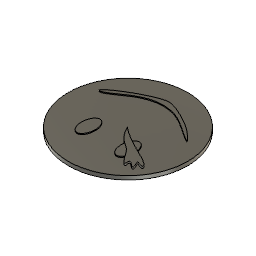
Comedian_Badge_v.1.0 (Autodesk Fusion 360 design; units mm, degrees)
part number: 2025-11-23-15-40-06-901
Autodesk Fusion 360 part; units mm, degrees
sketch "Sketch8" plane through (0, 0, 0) normal (0, 0, 1) x (1, 0, 0)
  circle A0 centre (0, 0) radius 73.66
  circle A1 centre (0, 0) radius 78.74
  arc A2 (-7.7116, -78.3615) -> (6.1475, -78.4997) centre (-0.7851, -78.7361) ccw
  arc A3 (-10.457, -78.213) -> (8.8953, -78.4059) centre (-0.7851, -78.7361) ccw
  dimension "d8" = 147.32
  dimension "d9" = 5.08
  dimension "d60" = 2.7495
  dimension "d61" = 78.7361
  dimension "d62" = 6.9366
  dimension "d63" = 0.5231
  constraint coincident A0.centre A1.centre
  constraint coincident A1 A2.centre
  constraint coincident A1 A2.start
  constraint coincident A1 A2.end
  measures "d8" diameter of A0
  measures "d61" vertical distance of A0.centre A2.centre
  measures "d62" radius of A2
  measures "d63" vertical distance of A2.centre A3.start
extrude "Inner Curve" add sketch "Sketch8" along normal blind 2.54 contours A0 makes body 1
extrude "Outer Curve" add sketch "Sketch8" along normal blind 5.08 from surface at -2.54 contours A1 bodies 1
sketch "Alignment 1" plane through (0, 0, 2.54) normal (0, 0, 1) x (-1, 0, 0)
  line L0 (0, 0) -> (52.0855, 52.0855) construction
  line L1 (0, 0) -> (-52.0855, 52.0855) construction
  line L2 (0, 0) -> (73.66, 0) construction
  line L3 (-26.0427, 26.0427) -> (26.0427, 26.0427) construction
  ellipse E0 centre (-26.0427, 26.0427) end of major axis (-26.0427, 41.2827) minor radius 8.89
  line L4 (-26.0427, 10.8027) -> (-26.0427, 41.2827) construction
  line L5 (-17.1527, 26.0427) -> (-34.9327, 26.0427) construction
  line L6 (0, 73.66) -> (0, -73.66) construction
  ellipse E1 centre (26.0427, 26.0427) end of major axis (26.0427, 41.2827) minor radius 8.89
  line L7 (0, 0) -> (0, -50.8) construction
  line L8 (34.9327, 26.0205) -> (34.9327, -64.8498) construction
  line L9 (-34.9327, 26.0427) -> (-34.9327, -64.2724) construction
  line L10 (-34.9327, -25.5899) -> (0, 0) construction
  line L11 (0, 0) -> (34.9327, -25.5899) construction
  circle A0 centre (0, 0) radius 78.74
  dimension "d16" = 73.66
  dimension "d17" = 135
  dimension "d18" = 73.66
  dimension "d19" = 30.48
  dimension "d20" = 17.78
  dimension "d23" = 50.8
  constraint coincident L0.start L1.start
  constraint horizontal L2
  constraint perpendicular L0 L1
  constraint midpoint L1 L3.start
  constraint midpoint L0 L3.end
  constraint coincident E0 L4.start
  constraint coincident E0 L4.end
  constraint coincident E0 L5.start
  constraint coincident E0 L5.end
  constraint coincident L3.start E0.centre
  constraint perpendicular L3 L4
  constraint perpendicular L2 L6
  constraint symmetric E0 L6 E1
  constraint coincident L3.end E1.centre
  constraint parallel L6 L7
  constraint coincident E1 L8.start
  constraint vertical L9
  constraint coincident L5.end L9.start
  constraint coincident L9 L10.start
  constraint symmetric L6 L10.start L11.end
  constraint coincident L8 L11.end
  measures "d16" distance of L0.start L0.end
  measures "d17" angle of L1 L2
  measures "d18" distance of L0.start L1.end
  measures "d19" distance of E0
  measures "d23" distance of L0.start L7.end
extrude "Eyes" add sketch "Alignment 1" along normal blind 1.27 contours E0 | E1 bodies 1
sketch "Alignment 2" plane through (0, 0, 2.54) normal (0, 0, 1) x (-1, 0, 0)
  ellipse E0 centre (26.0427, 26.0427) end of major axis (26.0427, 41.2827) minor radius 8.89
  ellipse E1 centre (-26.0427, 26.0427) end of major axis (-26.0427, 41.2827) minor radius 8.89
  line L0 (0.0807, 73.66) -> (0.0807, -73.66) construction
  line L1 (-34.9027, 24.7905) -> (-70.2813, -22.0531) construction
  line L2 (70.2813, -22.0531) -> (34.9327, 26.0427) construction
  line L3 (-70.2813, -22.0531) -> (70.2813, -22.0531) construction
  line L4 (70.2813, -22.0531) -> (-55.8551, -22.0531) construction
  line L5 (70.2813, -22.0531) -> (55.8541, -22.0531) construction
  circle A0 centre (0, 0) radius 78.74
  point P0 (70.2813, -22.0531)
  dimension "d25" = 140.5626
  dimension "d26" = 126.1364
  dimension "d27" = 14.4272
  dimension "d38" = 26.1235
  dimension "d40" = 37.062
  constraint vertical L0
  constraint coincident E1 L1.start
  constraint coincident E0 L2.end
  constraint horizontal L3
  constraint coincident P0 L2.start
  constraint parallel L3 L4
  constraint parallel L4 L5
  constraint horizontal E1.centre L2.end
  measures "d25" distance of L1.end P0
  measures "d26" distance of P0 L4.end
  measures "d27" distance of P0 L5.end
  measures "d38" distance of E1.centre L0
  measures "d40" angle of L0 L1
sketch "Blood Splatter" plane through (0, 0, 2.54) normal (0, 0, 1) x (-1, 0, 0)
  ellipse E0 centre (26.0427, 26.0427) end of major axis (26.0427, 41.2827) minor radius 8.89
  ellipse E1 centre (-26.0427, 26.0427) end of major axis (-26.0427, 41.2827) minor radius 8.89
  spline S0 degree 5 poles (0, 0) (0.1969, -0.2279) (0.5452, -0.589) (0.9093, -0.8334) (0.9612, -0.5275) (-0.05, 0.9191) (-2.4849, 3.3704) (-6.612, 6.7062) (-12.5588, 10.755) (-20.2217, 15.3044) (-29.241, 20.1083) (-38.8234, 24.9025) (-47.917, 29.3993) (-54.5396, 33.3328) (-57.6678, 36.3488) (-57.6761, 38.1034) (-55.5557, 38.4538) (-52.6453, 37.5711) (-50.0986, 36.1867) (-48.6444, 35.4193) (-48.5715, 36.1908) (-49.6251, 38.6476) (-51.0446, 41.8807) (-51.9382, 44.6253) (-51.5805, 45.747) (-49.7748, 44.8658) (-47.0902, 42.7681) (-44.4206, 40.7393) (-42.6094, 40.0043) (-42.0679, 41.1518) (-42.3499, 43.4995) (-42.6098, 45.7543) (-42.0762, 46.7002) (-40.6049, 45.9931) (-38.5035, 43.957) (-36.2304, 41.2005) (-34.0851, 38.2398) (-32.1418, 35.3844) (-30.3454, 32.8078) (-28.556, 30.5594) (-26.6153, 28.6009) (-24.4017, 26.8312) (-21.8967, 25.1168) (-19.1641, 23.3139) (-16.3177, 21.2902) (-13.4939, 18.9464) (-10.8205, 16.2389) (-8.3906, 13.1998) (-6.2268, 9.9645) (-4.3069, 6.7464) (-2.6019, 3.8005) (-1.4082, 1.8735) (-0.6359, 0.7782) (-0.1969, 0.2279) (0, 0) knots 0 0 0 0 0 0 0.02 0.04 0.06 0.08 0.1 0.12 0.14 0.16 0.18 0.2 0.22 0.24 0.26 0.28 0.3 0.32 0.34 0.36 0.38 0.4 0.42 0.44 0.46 0.48 0.5 0.52 0.54 0.56 0.58 0.6 0.62 0.64 0.66 0.68 0.7 0.72 0.74 0.76 0.78 0.8 0.82 0.84 0.86 0.88 0.9 0.92 0.94 0.96 0.98 1 1 1 1 1 1
  line L0 (-30.5379, 20.3586) -> (-61.7859, 36.9295)
  circle A0 centre (0, 0) radius 78.74
  point P0 (-46.1619, 28.644)
  point P1 (-53.9739, 37.8764)
  point P2 (-48.7659, 36.2193)
  point P3 (-51.3699, 45.215)
  point P4 (-42.8477, 40.4804)
  point P5 (-42.3742, 45.6884)
  point P6 (-37.6397, 42.8477)
  point P7 (-26.2768, 28.4073)
  point P8 (-10.416, 15.624)
  constraint coincident S0.start S0.end
  constraint midpoint P0 L0
extrude "Blood Splatter (1)" add sketch "Blood Splatter" along normal blind 2.54 separate body contours E1 S0 | E1 S0 | E1 S0 picked at (-25.5981, 21.049) picked at (-41.0519, 33.7718) picked at (-14.8563, 14.4402) makes body 2
sketch "Sketch18" plane through (0, 0, 2.54) normal (0, 0, 1) x (-1, 0, 0)
  spline S0 degree 5 poles (-55.9535, -21.9392) (-56.0022, -21.744) (-55.8793, -21.5301) (-55.0208, -21.7571) (-52.5792, -23.128) (-47.8442, -26.2124) (-42.0998, -30.0649) (-36.0544, -34.0423) (-30.3017, -37.604) (-25.1448, -40.4801) (-20.6388, -42.6257) (-16.6704, -44.1389) (-13.0259, -45.1898) (-9.4597, -45.9505) (-5.7724, -46.5104) (-1.8468, -46.8516) (2.3726, -46.8991) (6.8856, -46.5525) (11.6474, -45.7252) (16.5776, -44.3802) (21.5765, -42.5258) (26.5403, -40.2111) (31.3775, -37.5211) (36.0225, -34.5725) (40.457, -31.5086) (44.7078, -28.4957) (48.7877, -25.7179) (52.6437, -23.3733) (56.1063, -21.669) (58.8309, -20.8181) (60.2592, -21.0311) (59.9022, -22.4205) (57.6456, -24.8935) (53.6874, -28.2022) (48.4274, -32.0109) (42.3717, -35.9609) (36.0374, -39.7303) (29.8422, -43.1091) (24.0621, -46.0131) (18.8561, -48.4346) (14.2723, -50.4133) (10.2604, -51.9964) (6.6832, -53.2078) (3.3234, -54.0039) (-0.0891, -54.2677) (-3.8037, -53.8825) (-7.9919, -52.7801) (-12.6688, -51.0145) (-17.6745, -48.7761) (-22.7855, -46.2861) (-27.7875, -43.7268) (-32.5855, -41.1345) (-37.2462, -38.3635) (-42.2173, -34.8625) (-47.266, -30.8034) (-51.8146, -26.7345) (-54.4608, -24.0641) (-55.5866, -22.7015) (-55.9047, -22.1344) (-55.9535, -21.9392) knots 0 0 0 0 0 0 0.018182 0.036364 0.054545 0.072727 0.090909 0.109091 0.127273 0.145455 0.163636 0.181818 0.2 0.218182 0.236364 0.254545 0.272727 0.290909 0.309091 0.327273 0.345455 0.363636 0.381818 0.4 0.418182 0.436364 0.454545 0.472727 0.490909 0.509091 0.527273 0.545455 0.563636 0.581818 0.6 0.618182 0.636364 0.654545 0.672727 0.690909 0.709091 0.727273 0.745455 0.763636 0.781818 0.8 0.818182 0.836364 0.854545 0.872727 0.890909 0.909091 0.927273 0.945455 0.963636 0.981818 1 1 1 1 1 1
  line L0 (-23.2998, -46.7696) -> (-46.7696, -32.4836)
  point P0 (-35.2048, -34.5245)
  point P1 (-11.0546, -45.5791)
  point P2 (6.9729, -46.4295)
  point P3 (34.6946, -35.3748)
  point P4 (55.7834, -21.9392)
  point P5 (59.8651, -21.429)
  point P6 (39.2865, -37.7558)
  point P7 (7.9934, -52.7221)
  point P8 (-6.6328, -53.0623)
  point P9 (-35.0347, -39.6266)
  constraint midpoint P9 L0
extrude "Mouth" add sketch "Sketch18" along normal blind 1.27 bodies 1
